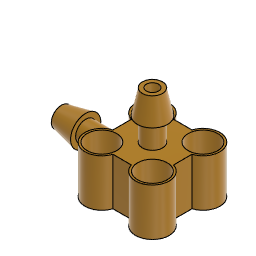
3P 2W Solenoid Valve Cap v23 (Autodesk Fusion 360 design; units mm, degrees)
Autodesk Fusion 360 part; units mm, degrees
note: some values were not read from the file. Chosen so that the rebuilt part matches the saved one: which bodies a step acts on; which face or edge a step refers to. Set by a fixed rule: which sketch regions a step uses.
sketch "Body Sketch" plane through (0, 0, 0) normal (0, 0, 1) x (1, 0, 0) in component "Cap"
  line L0 (-6.25, 6.25) -> (6.25, 6.25)
  line L1 (6.25, 6.25) -> (6.25, -6.25)
  line L2 (6.25, -6.25) -> (-6.25, -6.25)
  line L3 (-6.25, -6.25) -> (-6.25, 6.25)
  line L4 (-4.5, 4.5) -> (4.5, 4.5)
  line L5 (4.5, 4.5) -> (4.5, -4.5)
  line L6 (4.5, -4.5) -> (-4.5, -4.5)
  line L7 (-4.5, -4.5) -> (-4.5, 4.5)
  circle A0 centre (-3.75, 3.75) radius 2.5
  circle A1 centre (3.75, 3.75) radius 2.5
  circle A2 centre (3.75, -3.75) radius 2.5
  circle A3 centre (-3.75, -3.75) radius 2.5
  circle A4 centre (3.75, -3.75) radius 2.2
  circle A5 centre (-3.75, -3.75) radius 2.2
  circle A6 centre (-3.75, 3.75) radius 2.2
  circle A7 centre (3.75, 3.75) radius 2.2
  circle A8 centre (3.75, 3.75) radius 1.25
  circle A9 centre (3.75, -3.75) radius 1.25
  circle A10 centre (-3.75, -3.75) radius 1.25
  circle A11 centre (-3.75, 3.75) radius 1.25
  line L8 (-3.75, 3.75) -> (3.75, 3.75)
  line L9 (3.75, 3.75) -> (3.75, -3.75)
  line L10 (3.75, -3.75) -> (-3.75, -3.75)
  line L11 (-3.75, -3.75) -> (-3.75, 3.75)
  point P0 (0, 6.25)
  point P1 (6.25, 0)
  point P2 (0, 4.5)
  point P3 (4.5, 0)
  point P4 (-3.75, 0)
  point P5 (0, 3.75)
  dimension "d5" = 12.5
  dimension "d6" = 12.5
  dimension "d7" = 9
  dimension "d8" = 9
  dimension "d9" = 5
  dimension "d10" = 5
  dimension "d11" = 5
  dimension "d12" = 5
  dimension "d15" = 4.4
  dimension "d16" = 4.4
  dimension "d17" = 4.4
  dimension "d18" = 4.4
  dimension "d22" = 2.5
  dimension "d23" = 2.5
  dimension "d24" = 2.5
  dimension "d25" = 2.5
  dimension "d74" = 7.5
  dimension "d75" = 7.5
  constraint horizontal L0
  constraint vertical L1
  constraint horizontal L2
  constraint vertical L3
  constraint midpoint L0 P0
  constraint midpoint L1 P1
  constraint vertical origin P0
  constraint horizontal origin P1
  constraint horizontal L4
  constraint vertical L5
  constraint horizontal L6
  constraint vertical L7
  constraint midpoint L4 P2
  constraint midpoint L5 P3
  constraint vertical P0 P2
  constraint horizontal P1 P3
  constraint horizontal L8
  constraint vertical L9
  constraint horizontal L10
  constraint vertical L11
  constraint midpoint L11 P4
  constraint midpoint L8 P5
  constraint vertical P2 P5
  constraint horizontal P3 P4
  constraint coincident A1.centre A7.centre
  constraint coincident A3.centre A5.centre
  constraint coincident A2.centre A4.centre
  constraint coincident A0.centre A6.centre
  measures "d5" distance of L0.start L0.end
  measures "d6" distance of L0.start L2.end
  measures "d7" distance of L4.start L4.end
  measures "d8" distance of L4.start L6.end
  measures "d9" diameter of A0
  measures "d10" diameter of A1
  measures "d11" diameter of A2
  measures "d12" diameter of A3
  measures "d15" diameter of A4
  measures "d16" diameter of A5
  measures "d17" diameter of A6
  measures "d18" diameter of A7
  measures "d22" diameter of A8
  measures "d23" diameter of A9
  measures "d24" diameter of A10
  measures "d25" diameter of A11
  measures "d74" distance of A0.centre A1.centre
  measures "d75" distance of A0.centre A3.centre
extrude "Extrude9" add sketch "Body Sketch" against normal blind 7 contours L4 L7 A0 A6 | L4 L5 A1 A7 | L4 A0 A6 L8 | L6 L7 A3 A5 | L7 A0 A6 L11 | L4 A1 A7 L8 | L4 A6 A11 L8 | L4 L7 A6 A11 | A0 A6 L8 L11 | L7 A3 A5 L11 | L7 A6 A11 L11 | L5 L6 A2 A4 | L5 A1 A7 L9 | L4 L5 A7 A8 | L4 A7 A8 L8 | A1 A7 L8 L9 | A6 A11 L8 L11 | L7 A5 A10 L11 | L6 L7 A5 A10 | A3 A5 L10 L11 | L6 A3 A5 L10 | L5 A2 A4 L9 | L5 A7 A8 L9 | A7 A8 L8 L9 | A5 A10 L10 L11 | L6 A5 A10 L10 | L6 A2 A4 L10 | L5 L6 A4 A9 | L5 A4 A9 L9 | A2 A4 L9 L10 | L6 A4 A9 L10 | A4 A9 L9 L10 makes body 1 at (6.2376, -3.9989, -4.6667) makes body 2 at (-1.2624, -3.5011, -2.3333) makes body 3 at (6.2376, 3.5011, -4.6667) makes body 4 at (-1.2624, 3.9989, -2.3333) in component "Cap"
extrude "Extrude3" add sketch "Body Sketch" against normal blind 7 separate body contours L4 L7 A11 L8 L11 | L4 L7 A11 | L4 L5 A8 | L4 L5 A8 L8 L9 | A11 L8 L11 | L6 L7 A10 L10 L11 | L6 L7 A10 | A8 L8 L9 | A10 L10 L11 | L5 L6 A9 | L5 L6 A9 L9 L10 | A9 L9 L10 makes body 5 at (4.9938, 3.6255, -4.6667) makes body 6 at (4.9938, -3.8745, -4.6667) makes body 7 at (-2.5062, 3.6255, -4.6667) makes body 8 at (-2.5062, -3.8745, -4.6667) in component "Cap"
extrude "Extrude2" add sketch "Body Sketch" against normal blind 3.5 separate body contours L4 A6 A11 L8 | L4 L7 A6 A11 | L7 A6 A11 L11 | L4 L5 A7 A8 | L4 A7 A8 L8 | L4 L7 A11 L8 L11 | L4 L7 A11 | A6 A11 L8 L11 | L7 A5 A10 L11 | L6 L7 A5 A10 | L5 A7 A8 L9 | L4 L5 A8 | L4 L5 A8 L8 L9 | A7 A8 L8 L9 | A11 L8 L11 | L6 L7 A10 L10 L11 | L6 L7 A10 | A5 A10 L10 L11 | L6 A5 A10 L10 | L5 L6 A4 A9 | L5 A4 A9 L9 | A8 L8 L9 | A10 L10 L11 | L6 A4 A9 L10 | L5 L6 A9 | L5 L6 A9 L9 L10 | A4 A9 L9 L10 | A9 L9 L10 makes body 9 at (5.9391, -3.969, -2.3333) makes body 10 at (5.9391, 3.531, -2.3333) makes body 11 at (-1.5609, -3.531, -1.1667) makes body 12 at (-1.5609, 3.531, -2.3333) in component "Cap"
extrude "Extrude1" add sketch "Body Sketch" against normal blind 7 separate body contours L4 L7 A0 A6 | L4 L5 A1 A7 | L4 A0 A6 L8 | L4 A0 A1 L8 | L6 L7 A3 A5 | L7 A0 A3 L11 | L7 A0 A6 L11 | L4 A1 A7 L8 | L4 A6 A11 L8 | L4 L7 A6 A11 | A0 A1 A2 A3 L8 L9 L10 L11 | A0 A6 L8 L11 | L7 A3 A5 L11 | L7 A6 A11 L11 | L5 L6 A2 A4 | L5 A1 A7 L9 | L5 A1 A2 L9 | L4 L5 A7 A8 | L4 A7 A8 L8 | A1 A7 L8 L9 | L4 L7 A11 L8 L11 | L4 L7 A11 | A6 A11 L8 L11 | L7 A5 A10 L11 | L6 L7 A5 A10 | A3 A5 L10 L11 | L6 A2 A3 L10 | L6 A3 A5 L10 | L5 A2 A4 L9 | L5 A7 A8 L9 | L4 L5 A8 | L4 L5 A8 L8 L9 | A7 A8 L8 L9 | A11 L8 L11 | L6 L7 A10 L10 L11 | L6 L7 A10 | A5 A10 L10 L11 | L6 A5 A10 L10 | L6 A2 A4 L10 | L5 L6 A4 A9 | L5 A4 A9 L9 | A2 A4 L9 L10 | A8 L8 L9 | A10 L10 L11 | L6 A4 A9 L10 | L5 L6 A9 | L5 L6 A9 L9 L10 | A4 A9 L9 L10 | A9 L9 L10 makes body 13 in component "Cap"
combine "Combine1" operation cut target body 13 tool bodies 10 9 11 12 in component "Cap"
combine "Combine2" operation cut target body 13 tool bodies 6 8 7 5 in component "Cap"
sketch "Inner Chamber" plane through (0, 0, -7) normal (0, 0, -1) x (1, 0, 0) in component "Cap"
  circle A0 centre (3.75, -3.75) radius 1.25
  circle A1 centre (-3.75, -3.75) radius 1.25
  circle A2 centre (-3.75, 3.75) radius 1.25
  circle A3 centre (3.75, 3.75) radius 1.25
  arc A4 (1.3652, -4.5) -> (4.5, -1.3652) centre (3.75, -3.75) ccw
  line L0 (4.5, -1.3652) -> (4.5, 1.3652)
  arc A5 (4.5, 1.3652) -> (1.3652, 4.5) centre (3.75, 3.75) ccw
  line L1 (1.3652, 4.5) -> (-1.3652, 4.5)
  arc A6 (-1.3652, 4.5) -> (-4.5, 1.3652) centre (-3.75, 3.75) ccw
  line L2 (-4.5, 1.3652) -> (-4.5, -1.3652)
  arc A7 (-4.5, -1.3652) -> (-1.3652, -4.5) centre (-3.75, -3.75) ccw
  line L3 (-1.3652, -4.5) -> (1.3652, -4.5)
  circle A8 centre (0, 0) radius 3.25
  circle A9 centre (0, 0) radius 4
  dimension "d29" = 6.5
  dimension "d31" = 8
  constraint coincident A8.centre A9.centre
  measures "d29" diameter of A8
  measures "d31" diameter of A9
extrude "Extrude10" cut sketch "Inner Chamber" against normal blind 5.5 contours A8 keep common part bodies 1 2 3 4 in component "Cap"
extrude "Extrude5" cut sketch "Inner Chamber" against normal blind 0.75 contours A9 bodies 13 in component "Cap"
extrude "Extrude4" cut sketch "Inner Chamber" against normal blind 5.5 contours A8 bodies 13 in component "Cap"
sketch "Sketch3" plane through (0, -4.5, 0) normal (0, -1, 0) x (1, 0, 0) in component "Cap"
  line L0 (1.3652, 0) -> (-1.3652, 0)
  line L1 (-1.3652, 0) -> (-1.3652, -7)
  line L2 (-1.3652, -7) -> (1.3652, -7)
  line L3 (1.3652, -7) -> (1.3652, 0)
  point P0 (1.3652, -3.5)
  constraint midpoint L3 P0
sketch "Side Port (A)" plane through (0, 0, 0) normal (0, 1, 0) x (1, 0, 0) in component "Cap"
  line L0 (-4.5, 3.5) -> (-13.5, 3.5)
  line L1 (-13.5, 3.5) -> (-13.5, 2.5)
  line L2 (-13.5, 2.5) -> (-4.5, 2.5)
  line L3 (-4.5, 2.5) -> (-4.5, 3.5)
  line L4 (-4.5, 3.5) -> (-13.5, 3.5)
  line L5 (-13.5, 3.5) -> (-13.5, 2)
  line L6 (-13.5, 2) -> (-4.5, 2)
  line L7 (-4.5, 2) -> (-4.5, 3.5)
  line L8 (-13.5, 2) -> (-9.9, 2)
  line L9 (-9.9, 2) -> (-9.9, 1.25)
  line L10 (-9.9, 1.25) -> (-13.5, 2)
  point P0 (1.3652, 3.5)
  dimension "d45" = 9
  dimension "d46" = 1
  dimension "d47" = 1.5
  dimension "d48" = 3.6
  dimension "d51" = 0.75
  constraint horizontal L0
  constraint vertical L1
  constraint horizontal L2
  constraint vertical L3
  constraint horizontal L0.start P0
  constraint horizontal L4
  constraint vertical L5
  constraint horizontal L6
  constraint vertical L7
  constraint perpendicular L5 L8
  constraint perpendicular L6 L9
  constraint vertical L0.end L5.end
  measures "d45" distance of L0.start L0.end
  measures "d46" distance of L0.start L2.end
  measures "d47" distance of L0.start L6.end
  measures "d48" distance of L5.end L8.end
  measures "d51" distance of L8.end L9.end
revolve "Revolve1" add sketch "Side Port (A)" angle 360 about axis through (-4.5, 0, -3.5) along (-1, 0, 0) separate body contours L2 L5 L6 L7 L8 | L6 L8 L9 L10 makes body 14 in component "Cap"
sketch "Sketch5" plane through (-13.5, 0, 0) normal (-1, 0, 0) x (0, -1, 0) in component "Cap"
  circle A0 centre (0, -3.5) radius 1.5
  circle A1 centre (0, -3.5) radius 1
sketch "Sketch6" plane through (-4.5, 0, 0) normal (-1, 0, 0) x (0, -1, 0) in component "Cap"
  line L0 (1.3652, 0) -> (-1.3652, 0)
  line L1 (-1.3652, 0) -> (-1.3652, -7)
  line L2 (-1.3652, -7) -> (1.3652, -7)
  line L3 (1.3652, -7) -> (1.3652, 0)
  circle A0 centre (0, -3.5) radius 1.5
  circle A1 centre (0, -3.5) radius 1
extrude "Extrude6" cut sketch "Sketch6" against normal blind 2 contours A1 bodies 13 in component "Cap"
combine "Combine3" operation add target body 14 tool bodies 13 in component "Cap"
sketch "Top Port (" plane through (0, 0, 0) normal (0, 1, 0) x (1, 0, 0) in component "Cap"
  line L0 (0, 0) -> (0.9, 0)
  line L1 (0.9, 0) -> (0.9, -7)
  line L2 (0.9, -7) -> (0, -7)
  line L3 (0, -7) -> (0, 0)
  line L4 (0, 0) -> (1.5, 0)
  line L5 (1.5, 0) -> (1.5, -7)
  line L6 (1.5, -7) -> (0, -7)
  line L7 (0, -7) -> (0, 0)
  line L8 (1.5, -7) -> (1.5, -3.4)
  line L9 (1.5, -3.4) -> (2.25, -3.4)
  line L10 (2.25, -3.4) -> (1.5, -7)
  dimension "d60" = 0.9
  dimension "d61" = 7
  dimension "d62" = 1.5
  dimension "d63" = 7
  dimension "d64" = 3.6
  dimension "d65" = 0.75
  constraint horizontal L0
  constraint vertical L1
  constraint horizontal L2
  constraint vertical L3
  constraint coincident L0.start L3.end
  constraint horizontal L4
  constraint vertical L5
  constraint horizontal L6
  constraint vertical L7
  constraint perpendicular L6 L8
  constraint perpendicular L8 L9
  measures "d60" distance of L0.start L0.end
  measures "d61" distance of L0.start L2.end
  measures "d62" distance of L0.start L4.end
  measures "d63" distance of L0.start L2.end
  measures "d64" distance of L5.end L8.end
  measures "d65" distance of L8.end L9.end
revolve "Revolve2" add sketch "Top Port (" angle 360 about axis through (0, 0, 7) along (0, 0, -1) contours L1 L4 L5 L6 L8 | L5 L8 L9 L10 bodies 14 in component "Cap"
sketch "Sketch8" plane through (0, 0, -1.5) normal (0, 0, -1) x (1, 0, 0) in component "Cap"
  circle A0 centre (0, 0) radius 1.5
  circle A1 centre (0, 0) radius 0.9
  arc A2 (-1.8212, -2.6918) -> (-2.6918, -1.8212) centre (-3.75, -3.75) ccw
  arc A3 (-1.8212, -2.6918) -> (1.8212, -2.6918) centre (0, 0) ccw
  arc A4 (2.6918, -1.8212) -> (1.8212, -2.6918) centre (3.75, -3.75) ccw
  arc A5 (2.6918, -1.8212) -> (2.6918, 1.8212) centre (0, 0) ccw
  arc A6 (1.8212, 2.6918) -> (2.6918, 1.8212) centre (3.75, 3.75) ccw
  arc A7 (1.8212, 2.6918) -> (-1.8212, 2.6918) centre (0, 0) ccw
  arc A8 (-2.6918, 1.8212) -> (-1.8212, 2.6918) centre (-3.75, 3.75) ccw
  arc A9 (-2.6918, 1.8212) -> (-2.6918, -1.8212) centre (0, 0) ccw
extrude "Extrude7" add sketch "Sketch8" along normal blind 2 contours A0 bodies 14 in component "Cap"
extrude "Extrude8" cut 1 faces at (0.4737, 0.323, -1.5) along direction (0, 0, 1) blind 2 on bodies 14 bodies 14 in component "Cap"
combine "Combine4" operation add target body 4 tool bodies 3 2 1 makes body 15 at (-1.4221, -2.8384, -5.1667) makes body 16 at (1.4221, 2.8384, -3.3333) makes body 17 at (1.4221, -2.8384, -5.1667) in component "Cap"
combine "Combine5" operation add target body 14 tool bodies 17 15 16 4 in component "Cap"
extrude "Extrude11" cut sketch "Inner Chamber" against normal blind 2.75 contours A8 bodies 14 in component "Cap"
extrude "Extrude12" cut sketch "Body Sketch" against normal blind 3.5 contours L4 A6 A11 L8 | L4 L7 A6 A11 | L7 A6 A11 L11 | L4 L5 A7 A8 | L4 A7 A8 L8 | A6 A11 L8 L11 | L7 A5 A10 L11 | L6 L7 A5 A10 | L5 A7 A8 L9 | A7 A8 L8 L9 | A5 A10 L10 L11 | L6 A5 A10 L10 | L5 L6 A4 A9 | L5 A4 A9 L9 | L6 A4 A9 L10 | A4 A9 L9 L10 bodies 14 in component "Cap"
component "Cap" placed x (1, 0, 0) y (0, 1, 0) z (0, 0, 1) at (2, 0, 1)
component "References" placed x (1, 0, 0) y (0, 1, 0) z (0, 0, 1) at (0, 0, 0)
equation "Outter = 12.5 mm"
equation "Inner = 9 mm"
equation "Screw_d = 5 mm"
equation "Height = 7 mm"
equation "d5 = Outter"
equation "d6 = Outter"
equation "d7 = Inner"
equation "d8 = Inner"
equation "d9 = Screw_d"
equation "d10 = Screw_d"
equation "d11 = Screw_d"
equation "d12 = Screw_d"
equation "d13 = -Height"
equation "d15 = Screw_d - minWallThickness"
equation "d16 = Screw_d - minWallThickness"
equation "d17 = Screw_d - minWallThickness"
equation "d18 = Screw_d - minWallThickness"
equation "d19 = ( -Height / 2 mm ) * 1 mm"
equation "Screw_body = 2.5 mm"
equation "d22 = Screw_body"
equation "d23 = Screw_body"
equation "d24 = Screw_body"
equation "d25 = Screw_body"
equation "d26 = -Height"
equation "IN_Hole_d = 6.5 mm"
equation "d29 = IN_Hole_d"
equation "OD_Hole_d = 8 mm"
equation "d31 = OD_Hole_d"
equation "d32 = -InteriorChamber"
equation "InsulationRing_height = 0.75 mm"
equation "d35 = -InsulationRing_height"
equation "Standard_ID = 2 mm"
equation "Standard_OD = 4 mm"
equation "InteriorChamber = 5.5 mm"
equation "Barb_ID = 2 mm"
equation "Barb_length = 9 mm"
equation "Barb_OD = Barb_ID + 1 mm"
equation "d45 = Barb_length"
equation "d46 = Barb_ID / 2"
equation "d47 = Barb_OD / 2"
equation "d48 = Barb_FLength"
equation "Barb_FD = 4.5 mm"
equation "Barb_FE = Barb_FD - Barb_OD"
equation "d51 = Barb_FE / 2"
equation "TopBarb_ID = 1.8 mm"
equation "TopBarb_OD = 3 mm"
equation "TopBarb_FD = 4.5 mm"
equation "TopBarb_FE = TopBarb_FD - TopBarb_OD"
equation "TopBarb_length = 7 mm"
equation "d60 = TopBarb_ID / 2"
equation "d61 = TopBarb_length"
equation "d62 = TopBarb_OD / 2"
equation "d63 = TopBarb_length"
equation "d64 = TopBarb_FLength"
equation "d65 = TopBarb_FE / 2"
equation "TopBarb_innerLength = InteriorChamber - 3.5 mm"
equation "d68 = TopBarb_innerLength"
equation "d70 = ( Height - Inner )"
equation "minWallThickness = 0.6 mm"
equation "Screw_square = Outter - Screw_d"
equation "d74 = Screw_square"
equation "d75 = Screw_square"
equation "d76 = -Height"
equation "d78 = -InteriorChamber"
equation "d80 = -InteriorChamber / 2"
equation "d82 = -Height / 2"
equation "Barb_FLength = Barb_length * 4 / 10"
equation "TopBarb_FLength = Barb_length * 4 / 10"
named bodies: "Cap"
